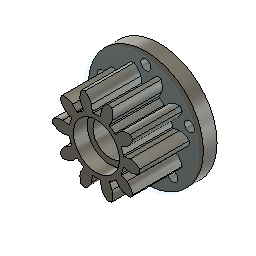
インナーギヤ v15 (Autodesk Fusion 360 design; units mm, degrees)
description: Spur Gear; Module: 1.580000; Num Teeth: 10; Pressure Angle: 20.000000; Backlash: 0.10 mm
Autodesk Fusion 360 part; units mm, degrees
(part 1 of 6)
sketch "スケッチ1" plane through (0, 0, 0) normal (0, 0, 1) x (1, 0, 0)
sketch "スケッチ2" plane through (0, 0, 0) normal (0, 0, -1) x (-1, 0, 0)
  circle A0 centre (0, 0) radius 5
  arc A1 (-5.434928, -4.325344) -> (-5.399704, -4.049062) centre (-5.559714, -4.169048) ccw
  line L0 (-5.434928, -4.325344) -> (-5.88157, -4.68194)
  spline S0 degree 5 poles (-5.88157, -4.68194) (-5.88496, -4.684646) (-5.891658, -4.690149) (-5.901465, -4.698676) (-5.914079, -4.710563) (-5.929217, -4.726135) (-5.943899, -4.742229) (-5.958299, -4.758658) (-5.972545, -4.775276) (-5.986688, -4.792027) (-6.000723, -4.808908) (-6.014614, -4.825957) (-6.028313, -4.84322) (-6.041787, -4.86073) (-6.05503, -4.87849) (-6.068059, -4.896482) (-6.080899, -4.914676) (-6.093581, -4.93304) (-6.106125, -4.951551) (-6.118538, -4.970199) (-6.13082, -4.988985) (-6.142963, -5.007914) (-6.15496, -5.026993) (-6.166806, -5.046226) (-6.178501, -5.06561) (-6.190051, -5.085142) (-6.20146, -5.104812) (-6.212734, -5.124615) (-6.22388, -5.144544) (-6.234897, -5.164595) (-6.245788, -5.184769) (-6.25655, -5.205064) (-6.267184, -5.225479) (-6.27769, -5.246016) (-6.288068, -5.266671) (-6.298319, -5.287442) (-6.308445, -5.308327) (-6.318449, -5.329324) (-6.32833, -5.35043) (-6.338091, -5.371643) (-6.347731, -5.392962) (-6.35725, -5.414386) (-6.36665, -5.435913) (-6.375931, -5.457544) (-6.385092, -5.479276) (-6.394135, -5.501107) (-6.40306, -5.523038) (-6.411868, -5.545065) (-6.420559, -5.567189) (-6.429134, -5.589407) (-6.437594, -5.611719) (-6.445937, -5.634123) (-6.454166, -5.656619) (-6.462279, -5.679205) (-6.470278, -5.701881) (-6.478163, -5.724646) (-6.485934, -5.747498) (-6.49359, -5.770436) (-6.501134, -5.79346) (-6.508564, -5.816568) (-6.515881, -5.839761) (-6.523086, -5.863036) (-6.530178, -5.886393) (-6.537157, -5.909831) (-6.544025, -5.93335) (-6.55078, -5.956947) (-6.557424, -5.980623) (-6.563955, -6.004376) (-6.570375, -6.028206) (-6.576684, -6.052112) (-6.582882, -6.076094) (-6.587751, -6.09534) (-6.591353, -6.109808) (-6.593732, -6.119468) (-6.594916, -6.124302) knots 0 0 0 0 0 0 0.01428571 0.02857143 0.04285714 0.05714286 0.07142857 0.08571429 0.1 0.11428571 0.12857143 0.14285714 0.15714286 0.17142857 0.18571429 0.2 0.21428571 0.22857143 0.24285714 0.25714286 0.27142857 0.28571429 0.3 0.31428571 0.32857143 0.34285714 0.35714286 0.37142857 0.38571429 0.4 0.41428571 0.42857143 0.44285714 0.45714286 0.47142857 0.48571429 0.5 0.51428571 0.52857143 0.54285714 0.55714286 0.57142857 0.58571429 0.6 0.61428571 0.62857143 0.64285714 0.65714286 0.67142857 0.68571429 0.7 0.71428571 0.72857143 0.74285714 0.75714286 0.77142857 0.78571429 0.8 0.81428571 0.82857143 0.84285714 0.85714286 0.87142857 0.88571429 0.9 0.91428571 0.92857143 0.94285714 0.95714286 0.97142857 0.98571429 1 1 1 1 1 1
  arc A2 (-6.594916, -6.124302) -> (-6.124302, -6.594916) centre (0, 0) ccw
  spline S1 degree 5 poles (-4.68194, -5.88157) (-4.684646, -5.88496) (-4.690149, -5.891658) (-4.698676, -5.901465) (-4.710563, -5.914079) (-4.726135, -5.929217) (-4.742229, -5.943899) (-4.758658, -5.958299) (-4.775276, -5.972545) (-4.792027, -5.986688) (-4.808908, -6.000723) (-4.825957, -6.014614) (-4.84322, -6.028313) (-4.86073, -6.041787) (-4.87849, -6.05503) (-4.896482, -6.068059) (-4.914676, -6.080899) (-4.93304, -6.093581) (-4.951551, -6.106125) (-4.970199, -6.118538) (-4.988985, -6.13082) (-5.007914, -6.142963) (-5.026993, -6.15496) (-5.046226, -6.166806) (-5.06561, -6.178501) (-5.085142, -6.190051) (-5.104812, -6.20146) (-5.124615, -6.212734) (-5.144544, -6.22388) (-5.164595, -6.234897) (-5.184769, -6.245788) (-5.205064, -6.25655) (-5.225479, -6.267184) (-5.246016, -6.27769) (-5.266671, -6.288068) (-5.287442, -6.298319) (-5.308327, -6.308445) (-5.329324, -6.318449) (-5.35043, -6.32833) (-5.371643, -6.338091) (-5.392962, -6.347731) (-5.414386, -6.35725) (-5.435913, -6.36665) (-5.457544, -6.375931) (-5.479276, -6.385092) (-5.501107, -6.394135) (-5.523038, -6.40306) (-5.545065, -6.411868) (-5.567189, -6.420559) (-5.589407, -6.429134) (-5.611719, -6.437594) (-5.634123, -6.445937) (-5.656619, -6.454166) (-5.679205, -6.462279) (-5.701881, -6.470278) (-5.724646, -6.478163) (-5.747498, -6.485934) (-5.770436, -6.49359) (-5.79346, -6.501134) (-5.816568, -6.508564) (-5.839761, -6.515881) (-5.863036, -6.523086) (-5.886393, -6.530178) (-5.909831, -6.537157) (-5.93335, -6.544025) (-5.956947, -6.55078) (-5.980623, -6.557424) (-6.004376, -6.563955) (-6.028206, -6.570375) (-6.052112, -6.576684) (-6.076094, -6.582882) (-6.09534, -6.587751) (-6.109808, -6.591353) (-6.119468, -6.593732) (-6.124302, -6.594916) knots 0 0 0 0 0 0 0.01428571 0.02857143 0.04285714 0.05714286 0.07142857 0.08571429 0.1 0.11428571 0.12857143 0.14285714 0.15714286 0.17142857 0.18571429 0.2 0.21428571 0.22857143 0.24285714 0.25714286 0.27142857 0.28571429 0.3 0.31428571 0.32857143 0.34285714 0.35714286 0.37142857 0.38571429 0.4 0.41428571 0.42857143 0.44285714 0.45714286 0.47142857 0.48571429 0.5 0.51428571 0.52857143 0.54285714 0.55714286 0.57142857 0.58571429 0.6 0.61428571 0.62857143 0.64285714 0.65714286 0.67142857 0.68571429 0.7 0.71428571 0.72857143 0.74285714 0.75714286 0.77142857 0.78571429 0.8 0.81428571 0.82857143 0.84285714 0.85714286 0.87142857 0.88571429 0.9 0.91428571 0.92857143 0.94285714 0.95714286 0.97142857 0.98571429 1 1 1 1 1 1
  line L1 (-4.68194, -5.88157) -> (-4.325344, -5.434928)
  arc A3 (-4.049062, -5.399704) -> (-4.325344, -5.434928) centre (-4.169048, -5.559714) ccw
  arc A4 (-4.049062, -5.399704) -> (-3.439167, -5.807222) centre (0, 0) ccw
  arc A5 (-3.365981, -6.075954) -> (-3.439167, -5.807222) centre (-3.54108, -5.979309) ccw
  line L2 (-3.365981, -6.075954) -> (-3.642161, -6.576327)
  spline S2 degree 5 poles (-3.642161, -6.576327) (-3.644257, -6.580125) (-3.64834, -6.587773) (-3.654137, -6.599403) (-3.661242, -6.615212) (-3.669269, -6.635392) (-3.676674, -6.655881) (-3.683691, -6.676569) (-3.690493, -6.697374) (-3.697149, -6.718261) (-3.703656, -6.739229) (-3.709965, -6.760296) (-3.716015, -6.781487) (-3.721762, -6.802821) (-3.727201, -6.824297) (-3.732353, -6.845905) (-3.737253, -6.867628) (-3.741942, -6.889448) (-3.746447, -6.91135) (-3.750779, -6.933329) (-3.754937, -6.955385) (-3.758912, -6.977519) (-3.762695, -6.999737) (-3.766279, -7.022039) (-3.769666, -7.044424) (-3.772862, -7.066888) (-3.775875, -7.089427) (-3.778713, -7.112037) (-3.781383, -7.134714) (-3.783889, -7.157456) (-3.78623, -7.180261) (-3.788407, -7.20313) (-3.790419, -7.226061) (-3.792266, -7.249054) (-3.79395, -7.272109) (-3.795472, -7.295222) (-3.796835, -7.318393) (-3.798041, -7.341619) (-3.799094, -7.3649) (-3.799994, -7.388233) (-3.800741, -7.411618) (-3.801338, -7.435054) (-3.801784, -7.458541) (-3.80208, -7.482076) (-3.802228, -7.505659) (-3.802228, -7.52929) (-3.802081, -7.552966) (-3.801789, -7.576688) (-3.801352, -7.600453) (-3.800772, -7.624262) (-3.800049, -7.648112) (-3.799184, -7.672004) (-3.798177, -7.695937) (-3.79703, -7.719909) (-3.795742, -7.74392) (-3.794315, -7.767969) (-3.792749, -7.792055) (-3.791045, -7.816177) (-3.789203, -7.840335) (-3.787225, -7.864528) (-3.78511, -7.888755) (-3.782859, -7.913015) (-3.780473, -7.937309) (-3.777952, -7.961634) (-3.775296, -7.98599) (-3.772507, -8.010377) (-3.769584, -8.034793) (-3.766529, -8.059237) (-3.763341, -8.08371) (-3.760021, -8.108211) (-3.756569, -8.132739) (-3.753703, -8.152383) (-3.751494, -8.167128) (-3.749995, -8.176964) (-3.749239, -8.181883) knots 0 0 0 0 0 0 0.01428571 0.02857143 0.04285714 0.05714286 0.07142857 0.08571429 0.1 0.11428571 0.12857143 0.14285714 0.15714286 0.17142857 0.18571429 0.2 0.21428571 0.22857143 0.24285714 0.25714286 0.27142857 0.28571429 0.3 0.31428571 0.32857143 0.34285714 0.35714286 0.37142857 0.38571429 0.4 0.41428571 0.42857143 0.44285714 0.45714286 0.47142857 0.48571429 0.5 0.51428571 0.52857143 0.54285714 0.55714286 0.57142857 0.58571429 0.6 0.61428571 0.62857143 0.64285714 0.65714286 0.67142857 0.68571429 0.7 0.71428571 0.72857143 0.74285714 0.75714286 0.77142857 0.78571429 0.8 0.81428571 0.82857143 0.84285714 0.85714286 0.87142857 0.88571429 0.9 0.91428571 0.92857143 0.94285714 0.95714286 0.97142857 0.98571429 1 1 1 1 1 1
  arc A6 (-3.749239, -8.181883) -> (-3.134352, -8.436577) centre (0, 0) ccw
  spline S3 degree 5 poles (-2.074769, -7.225563) (-2.075972, -7.22973) (-2.078493, -7.238025) (-2.082618, -7.250348) (-2.088772, -7.266551) (-2.097366, -7.286496) (-2.106617, -7.30622) (-2.116284, -7.32581) (-2.126186, -7.345331) (-2.136249, -7.364807) (-2.146475, -7.384235) (-2.15691, -7.403593) (-2.167616, -7.422855) (-2.178637, -7.442004) (-2.189978, -7.461035) (-2.201614, -7.479958) (-2.213509, -7.498784) (-2.225622, -7.517528) (-2.237924, -7.536201) (-2.250402, -7.554805) (-2.263058, -7.573341) (-2.275899, -7.591804) (-2.288935, -7.610188) (-2.30217, -7.628493) (-2.315604, -7.646716) (-2.329228, -7.66486) (-2.343036, -7.682929) (-2.357016, -7.700923) (-2.371163, -7.718847) (-2.385472, -7.736699) (-2.399942, -7.75448) (-2.414574, -7.77219) (-2.429366, -7.789828) (-2.444319, -7.807393) (-2.45943, -7.824885) (-2.474697, -7.842305) (-2.490117, -7.859653) (-2.505688, -7.876929) (-2.521405, -7.894135) (-2.537268, -7.911271) (-2.553276, -7.928335) (-2.569426, -7.945329) (-2.585717, -7.962252) (-2.60215, -7.979103) (-2.618722, -7.995884) (-2.635431, -8.012593) (-2.652276, -8.029231) (-2.669257, -8.045798) (-2.68637, -8.062294) (-2.703615, -8.078719) (-2.720992, -8.095073) (-2.738497, -8.111355) (-2.756132, -8.127566) (-2.773894, -8.143706) (-2.791783, -8.159773) (-2.809798, -8.175769) (-2.827936, -8.191694) (-2.846198, -8.207546) (-2.864583, -8.223326) (-2.883089, -8.239033) (-2.901715, -8.254669) (-2.920462, -8.270232) (-2.939327, -8.285723) (-2.95831, -8.30114) (-2.97741, -8.316485) (-2.996627, -8.331757) (-3.015958, -8.346955) (-3.035403, -8.362079) (-3.054963, -8.37713) (-3.074635, -8.392107) (-3.094419, -8.40701) (-3.110336, -8.418874) (-3.122325, -8.427738) (-3.130339, -8.433633) (-3.134352, -8.436577) knots 0 0 0 0 0 0 0.01428571 0.02857143 0.04285714 0.05714286 0.07142857 0.08571429 0.1 0.11428571 0.12857143 0.14285714 0.15714286 0.17142857 0.18571429 0.2 0.21428571 0.22857143 0.24285714 0.25714286 0.27142857 0.28571429 0.3 0.31428571 0.32857143 0.34285714 0.35714286 0.37142857 0.38571429 0.4 0.41428571 0.42857143 0.44285714 0.45714286 0.47142857 0.48571429 0.5 0.51428571 0.52857143 0.54285714 0.55714286 0.57142857 0.58571429 0.6 0.61428571 0.62857143 0.64285714 0.65714286 0.67142857 0.68571429 0.7 0.71428571 0.72857143 0.74285714 0.75714286 0.77142857 0.78571429 0.8 0.81428571 0.82857143 0.84285714 0.85714286 0.87142857 0.88571429 0.9 0.91428571 0.92857143 0.94285714 0.95714286 0.97142857 0.98571429 1 1 1 1 1 1
  line L3 (-2.074769, -7.225563) -> (-1.91624, -6.676457)
  arc A7 (-1.674468, -6.538185) -> (-1.91624, -6.676457) centre (-1.724088, -6.731931) ccw
  arc A8 (-1.674468, -6.538185) -> (-0.955048, -6.681286) centre (0, 0) ccw
  arc A9 (-0.784594, -6.901555) -> (-0.955048, -6.681286) centre (-0.983349, -6.879274) ccw
  line L4 (-0.784594, -6.901555) -> (-0.848267, -7.469529)
  spline S4 degree 5 poles (-0.848267, -7.469529) (-0.84875, -7.47384) (-0.849595, -7.482468) (-0.8505, -7.495431) (-0.851015, -7.512756) (-0.850708, -7.534471) (-0.849709, -7.556234) (-0.848274, -7.578033) (-0.846597, -7.599857) (-0.844753, -7.621702) (-0.84274, -7.643564) (-0.840507, -7.665441) (-0.837988, -7.687335) (-0.835133, -7.709243) (-0.831939, -7.731166) (-0.82843, -7.753101) (-0.824645, -7.775046) (-0.820626, -7.796999) (-0.816407, -7.818958) (-0.811998, -7.840922) (-0.807399, -7.86289) (-0.802601, -7.884861) (-0.797593, -7.906835) (-0.79237, -7.92881) (-0.786933, -7.950787) (-0.781289, -7.972765) (-0.775447, -7.994741) (-0.769417, -8.016717) (-0.763206, -8.038689) (-0.756818, -8.060658) (-0.750254, -8.082624) (-0.743513, -8.104585) (-0.736597, -8.126541) (-0.729504, -8.14849) (-0.722237, -8.170434) (-0.714798, -8.19237) (-0.70719, -8.214299) (-0.699417, -8.236219) (-0.69148, -8.25813) (-0.683382, -8.280032) (-0.675124, -8.301923) (-0.666706, -8.323804) (-0.65813, -8.345673) (-0.649398, -8.36753) (-0.640509, -8.389375) (-0.631466, -8.411206) (-0.62227, -8.433025) (-0.612922, -8.454829) (-0.603424, -8.476618) (-0.593777, -8.498392) (-0.583982, -8.52015) (-0.574039, -8.541893) (-0.563951, -8.563618) (-0.553717, -8.585326) (-0.543339, -8.607017) (-0.532817, -8.628689) (-0.522153, -8.650342) (-0.511347, -8.671976) (-0.500401, -8.693591) (-0.489315, -8.715185) (-0.47809, -8.736758) (-0.466726, -8.75831) (-0.455225, -8.779841) (-0.443587, -8.80135) (-0.431813, -8.822836) (-0.419903, -8.844299) (-0.40786, -8.865738) (-0.395682, -8.887153) (-0.383372, -8.908543) (-0.370928, -8.929908) (-0.358353, -8.951247) (-0.348188, -8.968299) (-0.340504, -8.981077) (-0.335355, -8.98959) (-0.332775, -8.993846) knots 0 0 0 0 0 0 0.01428571 0.02857143 0.04285714 0.05714286 0.07142857 0.08571429 0.1 0.11428571 0.12857143 0.14285714 0.15714286 0.17142857 0.18571429 0.2 0.21428571 0.22857143 0.24285714 0.25714286 0.27142857 0.28571429 0.3 0.31428571 0.32857143 0.34285714 0.35714286 0.37142857 0.38571429 0.4 0.41428571 0.42857143 0.44285714 0.45714286 0.47142857 0.48571429 0.5 0.51428571 0.52857143 0.54285714 0.55714286 0.57142857 0.58571429 0.6 0.61428571 0.62857143 0.64285714 0.65714286 0.67142857 0.68571429 0.7 0.71428571 0.72857143 0.74285714 0.75714286 0.77142857 0.78571429 0.8 0.81428571 0.82857143 0.84285714 0.85714286 0.87142857 0.88571429 0.9 0.91428571 0.92857143 0.94285714 0.95714286 0.97142857 0.98571429 1 1 1 1 1 1
  arc A10 (-0.332775, -8.993846) -> (0.332775, -8.993846) centre (0, 0) ccw
  spline S5 degree 5 poles (0.848267, -7.469529) (0.84875, -7.47384) (0.849595, -7.482468) (0.8505, -7.495431) (0.851015, -7.512756) (0.850708, -7.534471) (0.849709, -7.556234) (0.848274, -7.578033) (0.846597, -7.599857) (0.844753, -7.621702) (0.84274, -7.643564) (0.840507, -7.665441) (0.837988, -7.687335) (0.835133, -7.709243) (0.831939, -7.731166) (0.82843, -7.753101) (0.824645, -7.775046) (0.820626, -7.796999) (0.816407, -7.818958) (0.811998, -7.840922) (0.807399, -7.86289) (0.802601, -7.884861) (0.797593, -7.906835) (0.79237, -7.92881) (0.786933, -7.950787) (0.781289, -7.972765) (0.775447, -7.994741) (0.769417, -8.016717) (0.763206, -8.038689) (0.756818, -8.060658) (0.750254, -8.082624) (0.743513, -8.104585) (0.736597, -8.126541) (0.729504, -8.14849) (0.722237, -8.170434) (0.714798, -8.19237) (0.70719, -8.214299) (0.699417, -8.236219) (0.69148, -8.25813) (0.683382, -8.280032) (0.675124, -8.301923) (0.666706, -8.323804) (0.65813, -8.345673) (0.649398, -8.36753) (0.640509, -8.389375) (0.631466, -8.411206) (0.62227, -8.433025) (0.612922, -8.454829) (0.603424, -8.476618) (0.593777, -8.498392) (0.583982, -8.52015) (0.574039, -8.541893) (0.563951, -8.563618) (0.553717, -8.585326) (0.543339, -8.607017) (0.532817, -8.628689) (0.522153, -8.650342) (0.511347, -8.671976) (0.500401, -8.693591) (0.489315, -8.715185) (0.47809, -8.736758) (0.466726, -8.75831) (0.455225, -8.779841) (0.443587, -8.80135) (0.431813, -8.822836) (0.419903, -8.844299) (0.40786, -8.865738) (0.395682, -8.887153) (0.383372, -8.908543) (0.370928, -8.929908) (0.358353, -8.951247) (0.348188, -8.968299) (0.340504, -8.981077) (0.335355, -8.98959) (0.332775, -8.993846) knots 0 0 0 0 0 0 0.01428571 0.02857143 0.04285714 0.05714286 0.07142857 0.08571429 0.1 0.11428571 0.12857143 0.14285714 0.15714286 0.17142857 0.18571429 0.2 0.21428571 0.22857143 0.24285714 0.25714286 0.27142857 0.28571429 0.3 0.31428571 0.32857143 0.34285714 0.35714286 0.37142857 0.38571429 0.4 0.41428571 0.42857143 0.44285714 0.45714286 0.47142857 0.48571429 0.5 0.51428571 0.52857143 0.54285714 0.55714286 0.57142857 0.58571429 0.6 0.61428571 0.62857143 0.64285714 0.65714286 0.67142857 0.68571429 0.7 0.71428571 0.72857143 0.74285714 0.75714286 0.77142857 0.78571429 0.8 0.81428571 0.82857143 0.84285714 0.85714286 0.87142857 0.88571429 0.9 0.91428571 0.92857143 0.94285714 0.95714286 0.97142857 0.98571429 1 1 1 1 1 1
  line L5 (0.848267, -7.469529) -> (0.784594, -6.901555)
  arc A11 (0.955048, -6.681286) -> (0.784594, -6.901555) centre (0.983349, -6.879274) ccw
  arc A12 (0.955048, -6.681286) -> (1.674468, -6.538185) centre (0, 0) ccw
  arc A13 (1.91624, -6.676457) -> (1.674468, -6.538185) centre (1.724088, -6.731931) ccw
  line L6 (1.91624, -6.676457) -> (2.074769, -7.225563)
  spline S6 degree 5 poles (2.074769, -7.225563) (2.075972, -7.22973) (2.078493, -7.238025) (2.082618, -7.250348) (2.088772, -7.266551) (2.097366, -7.286496) (2.106617, -7.30622) (2.116284, -7.32581) (2.126186, -7.345331) (2.136249, -7.364807) (2.146475, -7.384235) (2.15691, -7.403593) (2.167616, -7.422855) (2.178637, -7.442004) (2.189978, -7.461035) (2.201614, -7.479958) (2.213509, -7.498784) (2.225622, -7.517528) (2.237924, -7.536201) (2.250402, -7.554805) (2.263058, -7.573341) (2.275899, -7.591804) (2.288935, -7.610188) (2.30217, -7.628493) (2.315604, -7.646716) (2.329228, -7.66486) (2.343036, -7.682929) (2.357016, -7.700923) (2.371163, -7.718847) (2.385472, -7.736699) (2.399942, -7.75448) (2.414574, -7.77219) (2.429366, -7.789828) (2.444319, -7.807393) (2.45943, -7.824885) (2.474697, -7.842305) (2.490117, -7.859653) (2.505688, -7.876929) (2.521405, -7.894135) (2.537268, -7.911271) (2.553276, -7.928335) (2.569426, -7.945329) (2.585717, -7.962252) (2.60215, -7.979103) (2.618722, -7.995884) (2.635431, -8.012593) (2.652276, -8.029231) (2.669257, -8.045798) (2.68637, -8.062294) (2.703615, -8.078719) (2.720992, -8.095073) (2.738497, -8.111355) (2.756132, -8.127566) (2.773894, -8.143706) (2.791783, -8.159773) (2.809798, -8.175769) (2.827936, -8.191694) (2.846198, -8.207546) (2.864583, -8.223326) (2.883089, -8.239033) (2.901715, -8.254669) (2.920462, -8.270232) (2.939327, -8.285723) (2.95831, -8.30114) (2.97741, -8.316485) (2.996627, -8.331757) (3.015958, -8.346955) (3.035403, -8.362079) (3.054963, -8.37713) (3.074635, -8.392107) (3.094419, -8.40701) (3.110336, -8.418874) (3.122325, -8.427738) (3.130339, -8.433633) (3.134352, -8.436577) knots 0 0 0 0 0 0 0.01428571 0.02857143 0.04285714 0.05714286 0.07142857 0.08571429 0.1 0.11428571 0.12857143 0.14285714 0.15714286 0.17142857 0.18571429 0.2 0.21428571 0.22857143 0.24285714 0.25714286 0.27142857 0.28571429 0.3 0.31428571 0.32857143 0.34285714 0.35714286 0.37142857 0.38571429 0.4 0.41428571 0.42857143 0.44285714 0.45714286 0.47142857 0.48571429 0.5 0.51428571 0.52857143 0.54285714 0.55714286 0.57142857 0.58571429 0.6 0.61428571 0.62857143 0.64285714 0.65714286 0.67142857 0.68571429 0.7 0.71428571 0.72857143 0.74285714 0.75714286 0.77142857 0.78571429 0.8 0.81428571 0.82857143 0.84285714 0.85714286 0.87142857 0.88571429 0.9 0.91428571 0.92857143 0.94285714 0.95714286 0.97142857 0.98571429 1 1 1 1 1 1
  arc A14 (3.134352, -8.436577) -> (3.749239, -8.181883) centre (0, 0) ccw
  spline S7 degree 5 poles (3.642161, -6.576327) (3.644257, -6.580125) (3.64834, -6.587773) (3.654137, -6.599403) (3.661242, -6.615212) (3.669269, -6.635392) (3.676674, -6.655881) (3.683691, -6.676569) (3.690493, -6.697374) (3.697149, -6.718261) (3.703656, -6.739229) (3.709965, -6.760296) (3.716015, -6.781487) (3.721762, -6.802821) (3.727201, -6.824297) (3.732353, -6.845905) (3.737253, -6.867628) (3.741942, -6.889448) (3.746447, -6.91135) (3.750779, -6.933329) (3.754937, -6.955385) (3.758912, -6.977519) (3.762695, -6.999737) (3.766279, -7.022039) (3.769666, -7.044424) (3.772862, -7.066888) (3.775875, -7.089427) (3.778713, -7.112037) (3.781383, -7.134714) (3.783889, -7.157456) (3.78623, -7.180261) (3.788407, -7.20313) (3.790419, -7.226061) (3.792266, -7.249054) (3.79395, -7.272109) (3.795472, -7.295222) (3.796835, -7.318393) (3.798041, -7.341619) (3.799094, -7.3649) (3.799994, -7.388233) (3.800741, -7.411618) (3.801338, -7.435054) (3.801784, -7.458541) (3.80208, -7.482076) (3.802228, -7.505659) (3.802228, -7.52929) (3.802081, -7.552966) (3.801789, -7.576688) (3.801352, -7.600453) (3.800772, -7.624262) (3.800049, -7.648112) (3.799184, -7.672004) (3.798177, -7.695937) (3.79703, -7.719909) (3.795742, -7.74392) (3.794315, -7.767969) (3.792749, -7.792055) (3.791045, -7.816177) (3.789203, -7.840335) (3.787225, -7.864528) (3.78511, -7.888755) (3.782859, -7.913015) (3.780473, -7.937309) (3.777952, -7.961634) (3.775296, -7.98599) (3.772507, -8.010377) (3.769584, -8.034793) (3.766529, -8.059237) (3.763341, -8.08371) (3.760021, -8.108211) (3.756569, -8.132739) (3.753703, -8.152383) (3.751494, -8.167128) (3.749995, -8.176964) (3.749239, -8.181883) knots 0 0 0 0 0 0 0.01428571 0.02857143 0.04285714 0.05714286 0.07142857 0.08571429 0.1 0.11428571 0.12857143 0.14285714 0.15714286 0.17142857 0.18571429 0.2 0.21428571 0.22857143 0.24285714 0.25714286 0.27142857 0.28571429 0.3 0.31428571 0.32857143 0.34285714 0.35714286 0.37142857 0.38571429 0.4 0.41428571 0.42857143 0.44285714 0.45714286 0.47142857 0.48571429 0.5 0.51428571 0.52857143 0.54285714 0.55714286 0.57142857 0.58571429 0.6 0.61428571 0.62857143 0.64285714 0.65714286 0.67142857 0.68571429 0.7 0.71428571 0.72857143 0.74285714 0.75714286 0.77142857 0.78571429 0.8 0.81428571 0.82857143 0.84285714 0.85714286 0.87142857 0.88571429 0.9 0.91428571 0.92857143 0.94285714 0.95714286 0.97142857 0.98571429 1 1 1 1 1 1
  line L7 (3.642161, -6.576327) -> (3.365981, -6.075954)
  arc A15 (3.439167, -5.807222) -> (3.365981, -6.075954) centre (3.54108, -5.979309) ccw
  arc A16 (3.439167, -5.807222) -> (4.049062, -5.399704) centre (0, 0) ccw
  arc A17 (4.325344, -5.434928) -> (4.049062, -5.399704) centre (4.169048, -5.559714) ccw
  line L8 (4.325344, -5.434928) -> (4.68194, -5.88157)
  spline S8 degree 5 poles (4.68194, -5.88157) (4.684646, -5.88496) (4.690149, -5.891658) (4.698676, -5.901465) (4.710563, -5.914079) (4.726135, -5.929217) (4.742229, -5.943899) (4.758658, -5.958299) (4.775276, -5.972545) (4.792027, -5.986688) (4.808908, -6.000723) (4.825957, -6.014614) (4.84322, -6.028313) (4.86073, -6.041787) (4.87849, -6.05503) (4.896482, -6.068059) (4.914676, -6.080899) (4.93304, -6.093581) (4.951551, -6.106125) (4.970199, -6.118538) (4.988985, -6.13082) (5.007914, -6.142963) (5.026993, -6.15496) (5.046226, -6.166806) (5.06561, -6.178501) (5.085142, -6.190051) (5.104812, -6.20146) (5.124615, -6.212734) (5.144544, -6.22388) (5.164595, -6.234897) (5.184769, -6.245788) (5.205064, -6.25655) (5.225479, -6.267184) (5.246016, -6.27769) (5.266671, -6.288068) (5.287442, -6.298319) (5.308327, -6.308445) (5.329324, -6.318449) (5.35043, -6.32833) (5.371643, -6.338091) (5.392962, -6.347731) (5.414386, -6.35725) (5.435913, -6.36665) (5.457544, -6.375931) (5.479276, -6.385092) (5.501107, -6.394135) (5.523038, -6.40306) (5.545065, -6.411868) (5.567189, -6.420559) (5.589407, -6.429134) (5.611719, -6.437594) (5.634123, -6.445937) (5.656619, -6.454166) (5.679205, -6.462279) (5.701881, -6.470278) (5.724646, -6.478163) (5.747498, -6.485934) (5.770436, -6.49359) (5.79346, -6.501134) (5.816568, -6.508564) (5.839761, -6.515881) (5.863036, -6.523086) (5.886393, -6.530178) (5.909831, -6.537157) (5.93335, -6.544025) (5.956947, -6.55078) (5.980623, -6.557424) (6.004376, -6.563955) (6.028206, -6.570375) (6.052112, -6.576684) (6.076094, -6.582882) (6.09534, -6.587751) (6.109808, -6.591353) (6.119468, -6.593732) (6.124302, -6.594916) knots 0 0 0 0 0 0 0.01428571 0.02857143 0.04285714 0.05714286 0.07142857 0.08571429 0.1 0.11428571 0.12857143 0.14285714 0.15714286 0.17142857 0.18571429 0.2 0.21428571 0.22857143 0.24285714 0.25714286 0.27142857 0.28571429 0.3 0.31428571 0.32857143 0.34285714 0.35714286 0.37142857 0.38571429 0.4 0.41428571 0.42857143 0.44285714 0.45714286 0.47142857 0.48571429 0.5 0.51428571 0.52857143 0.54285714 0.55714286 0.57142857 0.58571429 0.6 0.61428571 0.62857143 0.64285714 0.65714286 0.67142857 0.68571429 0.7 0.71428571 0.72857143 0.74285714 0.75714286 0.77142857 0.78571429 0.8 0.81428571 0.82857143 0.84285714 0.85714286 0.87142857 0.88571429 0.9 0.91428571 0.92857143 0.94285714 0.95714286 0.97142857 0.98571429 1 1 1 1 1 1
  arc A18 (6.124302, -6.594916) -> (6.594916, -6.124302) centre (0, 0) ccw
  spline S9 degree 5 poles (5.88157, -4.68194) (5.88496, -4.684646) (5.891658, -4.690149) (5.901465, -4.698676) (5.914079, -4.710563) (5.929217, -4.726135) (5.943899, -4.742229) (5.958299, -4.758658) (5.972545, -4.775276) (5.986688, -4.792027) (6.000723, -4.808908) (6.014614, -4.825957) (6.028313, -4.84322) (6.041787, -4.86073) (6.05503, -4.87849) (6.068059, -4.896482) (6.080899, -4.914676) (6.093581, -4.93304) (6.106125, -4.951551) (6.118538, -4.970199) (6.13082, -4.988985) (6.142963, -5.007914) (6.15496, -5.026993) (6.166806, -5.046226) (6.178501, -5.06561) (6.190051, -5.085142) (6.20146, -5.104812) (6.212734, -5.124615) (6.22388, -5.144544) (6.234897, -5.164595) (6.245788, -5.184769) (6.25655, -5.205064) (6.267184, -5.225479) (6.27769, -5.246016) (6.288068, -5.266671) (6.298319, -5.287442) (6.308445, -5.308327) (6.318449, -5.329324) (6.32833, -5.35043) (6.338091, -5.371643) (6.347731, -5.392962) (6.35725, -5.414386) (6.36665, -5.435913) (6.375931, -5.457544) (6.385092, -5.479276) (6.394135, -5.501107) (6.40306, -5.523038) (6.411868, -5.545065) (6.420559, -5.567189) (6.429134, -5.589407) (6.437594, -5.611719) (6.445937, -5.634123) (6.454166, -5.656619) (6.462279, -5.679205) (6.470278, -5.701881) (6.478163, -5.724646) (6.485934, -5.747498) (6.49359, -5.770436) (6.501134, -5.79346) (6.508564, -5.816568) (6.515881, -5.839761) (6.523086, -5.863036) (6.530178, -5.886393) (6.537157, -5.909831) (6.544025, -5.93335) (6.55078, -5.956947) (6.557424, -5.980623) (6.563955, -6.004376) (6.570375, -6.028206) (6.576684, -6.052112) (6.582882, -6.076094) (6.587751, -6.09534) (6.591353, -6.109808) (6.593732, -6.119468) (6.594916, -6.124302) knots 0 0 0 0 0 0 0.01428571 0.02857143 0.04285714 0.05714286 0.07142857 0.08571429 0.1 0.11428571 0.12857143 0.14285714 0.15714286 0.17142857 0.18571429 0.2 0.21428571 0.22857143 0.24285714 0.25714286 0.27142857 0.28571429 0.3 0.31428571 0.32857143 0.34285714 0.35714286 0.37142857 0.38571429 0.4 0.41428571 0.42857143 0.44285714 0.45714286 0.47142857 0.48571429 0.5 0.51428571 0.52857143 0.54285714 0.55714286 0.57142857 0.58571429 0.6 0.61428571 0.62857143 0.64285714 0.65714286 0.67142857 0.68571429 0.7 0.71428571 0.72857143 0.74285714 0.75714286 0.77142857 0.78571429 0.8 0.81428571 0.82857143 0.84285714 0.85714286 0.87142857 0.88571429 0.9 0.91428571 0.92857143 0.94285714 0.95714286 0.97142857 0.98571429 1 1 1 1 1 1
  line L9 (5.88157, -4.68194) -> (5.434928, -4.325344)
  arc A19 (5.399704, -4.049062) -> (5.434928, -4.325344) centre (5.559714, -4.169048) ccw
  arc A20 (5.399704, -4.049062) -> (5.807222, -3.439167) centre (0, 0) ccw
  arc A21 (6.075954, -3.365981) -> (5.807222, -3.439167) centre (5.979309, -3.54108) ccw
  line L10 (6.075954, -3.365981) -> (6.576327, -3.642161)
  spline S10 degree 5 poles (6.576327, -3.642161) (6.580125, -3.644257) (6.587773, -3.64834) (6.599403, -3.654137) (6.615212, -3.661242) (6.635392, -3.669269) (6.655881, -3.676674) (6.676569, -3.683691) (6.697374, -3.690493) (6.718261, -3.697149) (6.739229, -3.703656) (6.760296, -3.709965) (6.781487, -3.716015) (6.802821, -3.721762) (6.824297, -3.727201) (6.845905, -3.732353) (6.867628, -3.737253) (6.889448, -3.741942) (6.91135, -3.746447) (6.933329, -3.750779) (6.955385, -3.754937) (6.977519, -3.758912) (6.999737, -3.762695) (7.022039, -3.766279) (7.044424, -3.769666) (7.066888, -3.772862) (7.089427, -3.775875) (7.112037, -3.778713) (7.134714, -3.781383) (7.157456, -3.783889) (7.180261, -3.78623) (7.20313, -3.788407) (7.226061, -3.790419) (7.249054, -3.792266) (7.272109, -3.79395) (7.295222, -3.795472) (7.318393, -3.796835) (7.341619, -3.798041) (7.3649, -3.799094) (7.388233, -3.799994) (7.411618, -3.800741) (7.435054, -3.801338) (7.458541, -3.801784) (7.482076, -3.80208) (7.505659, -3.802228) (7.52929, -3.802228) (7.552966, -3.802081) (7.576688, -3.801789) (7.600453, -3.801352) (7.624262, -3.800772) (7.648112, -3.800049) (7.672004, -3.799184) (7.695937, -3.798177) (7.719909, -3.79703) (7.74392, -3.795742) (7.767969, -3.794315) (7.792055, -3.792749) (7.816177, -3.791045) (7.840335, -3.789203) (7.864528, -3.787225) (7.888755, -3.78511) (7.913015, -3.782859) (7.937309, -3.780473) (7.961634, -3.777952) (7.98599, -3.775296) (8.010377, -3.772507) (8.034793, -3.769584) (8.059237, -3.766529) (8.08371, -3.763341) (8.108211, -3.760021) (8.132739, -3.756569) (8.152383, -3.753703) (8.167128, -3.751494) (8.176964, -3.749995) (8.181883, -3.749239) knots 0 0 0 0 0 0 0.01428571 0.02857143 0.04285714 0.05714286 0.07142857 0.08571429 0.1 0.11428571 0.12857143 0.14285714 0.15714286 0.17142857 0.18571429 0.2 0.21428571 0.22857143 0.24285714 0.25714286 0.27142857 0.28571429 0.3 0.31428571 0.32857143 0.34285714 0.35714286 0.37142857 0.38571429 0.4 0.41428571 0.42857143 0.44285714 0.45714286 0.47142857 0.48571429 0.5 0.51428571 0.52857143 0.54285714 0.55714286 0.57142857 0.58571429 0.6 0.61428571 0.62857143 0.64285714 0.65714286 0.67142857 0.68571429 0.7 0.71428571 0.72857143 0.74285714 0.75714286 0.77142857 0.78571429 0.8 0.81428571 0.82857143 0.84285714 0.85714286 0.87142857 0.88571429 0.9 0.91428571 0.92857143 0.94285714 0.95714286 0.97142857 0.98571429 1 1 1 1 1 1
  arc A22 (8.181883, -3.749239) -> (8.436577, -3.134352) centre (0, 0) ccw
  spline S11 degree 5 poles (7.225563, -2.074769) (7.22973, -2.075972) (7.238025, -2.078493) (7.250348, -2.082618) (7.266551, -2.088772) (7.286496, -2.097366) (7.30622, -2.106617) (7.32581, -2.116284) (7.345331, -2.126186) (7.364807, -2.136249) (7.384235, -2.146475) (7.403593, -2.15691) (7.422855, -2.167616) (7.442004, -2.178637) (7.461035, -2.189978) (7.479958, -2.201614) (7.498784, -2.213509) (7.517528, -2.225622) (7.536201, -2.237924) (7.554805, -2.250402) (7.573341, -2.263058) (7.591804, -2.275899) (7.610188, -2.288935) (7.628493, -2.30217) (7.646716, -2.315604) (7.66486, -2.329228) (7.682929, -2.343036) (7.700923, -2.357016) (7.718847, -2.371163) (7.736699, -2.385472) (7.75448, -2.399942) (7.77219, -2.414574) (7.789828, -2.429366) (7.807393, -2.444319) (7.824885, -2.45943) (7.842305, -2.474697) (7.859653, -2.490117) (7.876929, -2.505688) (7.894135, -2.521405) (7.911271, -2.537268) (7.928335, -2.553276) (7.945329, -2.569426) (7.962252, -2.585717) (7.979103, -2.60215) (7.995884, -2.618722) (8.012593, -2.635431) (8.029231, -2.652276) (8.045798, -2.669257) (8.062294, -2.68637) (8.078719, -2.703615) (8.095073, -2.720992) (8.111355, -2.738497) (8.127566, -2.756132) (8.143706, -2.773894) (8.159773, -2.791783) (8.175769, -2.809798) (8.191694, -2.827936) (8.207546, -2.846198) (8.223326, -2.864583) (8.239033, -2.883089) (8.254669, -2.901715) (8.270232, -2.920462) (8.285723, -2.939327) (8.30114, -2.95831) (8.316485, -2.97741) (8.331757, -2.996627) (8.346955, -3.015958) (8.362079, -3.035403) (8.37713, -3.054963) (8.392107, -3.074635) (8.40701, -3.094419) (8.418874, -3.110336) (8.427738, -3.122325) (8.433633, -3.130339) (8.436577, -3.134352) knots 0 0 0 0 0 0 0.01428571 0.02857143 0.04285714 0.05714286 0.07142857 0.08571429 0.1 0.11428571 0.12857143 0.14285714 0.15714286 0.17142857 0.18571429 0.2 0.21428571 0.22857143 0.24285714 0.25714286 0.27142857 0.28571429 0.3 0.31428571 0.32857143 0.34285714 0.35714286 0.37142857 0.38571429 0.4 0.41428571 0.42857143 0.44285714 0.45714286 0.47142857 0.48571429 0.5 0.51428571 0.52857143 0.54285714 0.55714286 0.57142857 0.58571429 0.6 0.61428571 0.62857143 0.64285714 0.65714286 0.67142857 0.68571429 0.7 0.71428571 0.72857143 0.74285714 0.75714286 0.77142857 0.78571429 0.8 0.81428571 0.82857143 0.84285714 0.85714286 0.87142857 0.88571429 0.9 0.91428571 0.92857143 0.94285714 0.95714286 0.97142857 0.98571429 1 1 1 1 1 1
  line L11 (7.225563, -2.074769) -> (6.676457, -1.91624)
  arc A23 (6.538185, -1.674468) -> (6.676457, -1.91624) centre (6.731931, -1.724088) ccw
  arc A24 (6.538185, -1.674468) -> (6.681286, -0.955048) centre (0, 0) ccw
  arc A25 (6.901555, -0.784594) -> (6.681286, -0.955048) centre (6.879274, -0.983349) ccw
  line L12 (6.901555, -0.784594) -> (7.469529, -0.848267)
  spline S12 degree 5 poles (7.469529, -0.848267) (7.47384, -0.84875) (7.482468, -0.849595) (7.495431, -0.8505) (7.512756, -0.851015) (7.534471, -0.850708) (7.556234, -0.849709) (7.578033, -0.848274) (7.599857, -0.846597) (7.621702, -0.844753) (7.643564, -0.84274) (7.665441, -0.840507) (7.687335, -0.837988) (7.709243, -0.835133) (7.731166, -0.831939) (7.753101, -0.82843) (7.775046, -0.824645) (7.796999, -0.820626) (7.818958, -0.816407) (7.840922, -0.811998) (7.86289, -0.807399) (7.884861, -0.802601) (7.906835, -0.797593) (7.92881, -0.79237) (7.950787, -0.786933) (7.972765, -0.781289) (7.994741, -0.775447) (8.016717, -0.769417) (8.038689, -0.763206) (8.060658, -0.756818) (8.082624, -0.750254) (8.104585, -0.743513) (8.126541, -0.736597) (8.14849, -0.729504) (8.170434, -0.722237) (8.19237, -0.714798) (8.214299, -0.70719) (8.236219, -0.699417) (8.25813, -0.69148) (8.280032, -0.683382) (8.301923, -0.675124) (8.323804, -0.666706) (8.345673, -0.65813) (8.36753, -0.649398) (8.389375, -0.640509) (8.411206, -0.631466) (8.433025, -0.62227) (8.454829, -0.612922) (8.476618, -0.603424) (8.498392, -0.593777) (8.52015, -0.583982) (8.541893, -0.574039) (8.563618, -0.563951) (8.585326, -0.553717) (8.607017, -0.543339) (8.628689, -0.532817) (8.650342, -0.522153) (8.671976, -0.511347) (8.693591, -0.500401) (8.715185, -0.489315) (8.736758, -0.47809) (8.75831, -0.466726) (8.779841, -0.455225) (8.80135, -0.443587) (8.822836, -0.431813) (8.844299, -0.419903) (8.865738, -0.40786) (8.887153, -0.395682) (8.908543, -0.383372) (8.929908, -0.370928) (8.951247, -0.358353) (8.968299, -0.348188) (8.981077, -0.340504) (8.98959, -0.335355) (8.993846, -0.332775) knots 0 0 0 0 0 0 0.01428571 0.02857143 0.04285714 0.05714286 0.07142857 0.08571429 0.1 0.11428571 0.12857143 0.14285714 0.15714286 0.17142857 0.18571429 0.2 0.21428571 0.22857143 0.24285714 0.25714286 0.27142857 0.28571429 0.3 0.31428571 0.32857143 0.34285714 0.35714286 0.37142857 0.38571429 0.4 0.41428571 0.42857143 0.44285714 0.45714286 0.47142857 0.48571429 0.5 0.51428571 0.52857143 0.54285714 0.55714286 0.57142857 0.58571429 0.6 0.61428571 0.62857143 0.64285714 0.65714286 0.67142857 0.68571429 0.7 0.71428571 0.72857143 0.74285714 0.75714286 0.77142857 0.78571429 0.8 0.81428571 0.82857143 0.84285714 0.85714286 0.87142857 0.88571429 0.9 0.91428571 0.92857143 0.94285714 0.95714286 0.97142857 0.98571429 1 1 1 1 1 1
  arc A26 (8.993846, -0.332775) -> (8.993846, 0.332775) centre (0, 0) ccw
  spline S13 degree 5 poles (7.469529, 0.848267) (7.47384, 0.84875) (7.482468, 0.849595) (7.495431, 0.8505) (7.512756, 0.851015) (7.534471, 0.850708) (7.556234, 0.849709) (7.578033, 0.848274) (7.599857, 0.846597) (7.621702, 0.844753) (7.643564, 0.84274) (7.665441, 0.840507) (7.687335, 0.837988) (7.709243, 0.835133) (7.731166, 0.831939) (7.753101, 0.82843) (7.775046, 0.824645) (7.796999, 0.820626) (7.818958, 0.816407) (7.840922, 0.811998) (7.86289, 0.807399) (7.884861, 0.802601) (7.906835, 0.797593) (7.92881, 0.79237) (7.950787, 0.786933) (7.972765, 0.781289) (7.994741, 0.775447) (8.016717, 0.769417) (8.038689, 0.763206) (8.060658, 0.756818) (8.082624, 0.750254) (8.104585, 0.743513) (8.126541, 0.736597) (8.14849, 0.729504) (8.170434, 0.722237) (8.19237, 0.714798) (8.214299, 0.70719) (8.236219, 0.699417) (8.25813, 0.69148) (8.280032, 0.683382) (8.301923, 0.675124) (8.323804, 0.666706) (8.345673, 0.65813) (8.36753, 0.649398) (8.389375, 0.640509) (8.411206, 0.631466) (8.433025, 0.62227) (8.454829, 0.612922) (8.476618, 0.603424) (8.498392, 0.593777) (8.52015, 0.583982) (8.541893, 0.574039) (8.563618, 0.563951) (8.585326, 0.553717) (8.607017, 0.543339) (8.628689, 0.532817) (8.650342, 0.522153) (8.671976, 0.511347) (8.693591, 0.500401) (8.715185, 0.489315) (8.736758, 0.47809) (8.75831, 0.466726) (8.779841, 0.455225) (8.80135, 0.443587) (8.822836, 0.431813) (8.844299, 0.419903) (8.865738, 0.40786) (8.887153, 0.395682) (8.908543, 0.383372) (8.929908, 0.370928) (8.951247, 0.358353) (8.968299, 0.348188) (8.981077, 0.340504) (8.98959, 0.335355) (8.993846, 0.332775) knots 0 0 0 0 0 0 0.01428571 0.02857143 0.04285714 0.05714286 0.07142857 0.08571429 0.1 0.11428571 0.12857143 0.14285714 0.15714286 0.17142857 0.18571429 0.2 0.21428571 0.22857143 0.24285714 0.25714286 0.27142857 0.28571429 0.3 0.31428571 0.32857143 0.34285714 0.35714286 0.37142857 0.38571429 0.4 0.41428571 0.42857143 0.44285714 0.45714286 0.47142857 0.48571429 0.5 0.51428571 0.52857143 0.54285714 0.55714286 0.57142857 0.58571429 0.6 0.61428571 0.62857143 0.64285714 0.65714286 0.67142857 0.68571429 0.7 0.71428571 0.72857143 0.74285714 0.75714286 0.77142857 0.78571429 0.8 0.81428571 0.82857143 0.84285714 0.85714286 0.87142857 0.88571429 0.9 0.91428571 0.92857143 0.94285714 0.95714286 0.97142857 0.98571429 1 1 1 1 1 1
  line L13 (7.469529, 0.848267) -> (6.901555, 0.784594)
  arc A27 (6.681286, 0.955048) -> (6.901555, 0.784594) centre (6.879274, 0.983349) ccw
  arc A28 (6.681286, 0.955048) -> (6.538185, 1.674468) centre (0, 0) ccw
  arc A29 (6.676457, 1.91624) -> (6.538185, 1.674468) centre (6.731931, 1.724088) ccw
  line L14 (6.676457, 1.91624) -> (7.225563, 2.074769)
  spline S14 degree 5 poles (7.225563, 2.074769) (7.22973, 2.075972) (7.238025, 2.078493) (7.250348, 2.082618) (7.266551, 2.088772) (7.286496, 2.097366) (7.30622, 2.106617) (7.32581, 2.116284) (7.345331, 2.126186) (7.364807, 2.136249) (7.384235, 2.146475) (7.403593, 2.15691) (7.422855, 2.167616) (7.442004, 2.178637) (7.461035, 2.189978) (7.479958, 2.201614) (7.498784, 2.213509) (7.517528, 2.225622) (7.536201, 2.237924) (7.554805, 2.250402) (7.573341, 2.263058) (7.591804, 2.275899) (7.610188, 2.288935) (7.628493, 2.30217) (7.646716, 2.315604) (7.66486, 2.329228) (7.682929, 2.343036) (7.700923, 2.357016) (7.718847, 2.371163) (7.736699, 2.385472) (7.75448, 2.399942) (7.77219, 2.414574) (7.789828, 2.429366) (7.807393, 2.444319) (7.824885, 2.45943) (7.842305, 2.474697) (7.859653, 2.490117) (7.876929, 2.505688) (7.894135, 2.521405) (7.911271, 2.537268) (7.928335, 2.553276) (7.945329, 2.569426) (7.962252, 2.585717) (7.979103, 2.60215) (7.995884, 2.618722) (8.012593, 2.635431) (8.029231, 2.652276) (8.045798, 2.669257) (8.062294, 2.68637) (8.078719, 2.703615) (8.095073, 2.720992) (8.111355, 2.738497) (8.127566, 2.756132) (8.143706, 2.773894) (8.159773, 2.791783) (8.175769, 2.809798) (8.191694, 2.827936) (8.207546, 2.846198) (8.223326, 2.864583) (8.239033, 2.883089) (8.254669, 2.901715) (8.270232, 2.920462) (8.285723, 2.939327) (8.30114, 2.95831) (8.316485, 2.97741) (8.331757, 2.996627) (8.346955, 3.015958) (8.362079, 3.035403) (8.37713, 3.054963) (8.392107, 3.074635) (8.40701, 3.094419) (8.418874, 3.110336) (8.427738, 3.122325) (8.433633, 3.130339) (8.436577, 3.134352) knots 0 0 0 0 0 0 0.01428571 0.02857143 0.04285714 0.05714286 0.07142857 0.08571429 0.1 0.11428571 0.12857143 0.14285714 0.15714286 0.17142857 0.18571429 0.2 0.21428571 0.22857143 0.24285714 0.25714286 0.27142857 0.28571429 0.3 0.31428571 0.32857143 0.34285714 0.35714286 0.37142857 0.38571429 0.4 0.41428571 0.42857143 0.44285714 0.45714286 0.47142857 0.48571429 0.5 0.51428571 0.52857143 0.54285714 0.55714286 0.57142857 0.58571429 0.6 0.61428571 0.62857143 0.64285714 0.65714286 0.67142857 0.68571429 0.7 0.71428571 0.72857143 0.74285714 0.75714286 0.77142857 0.78571429 0.8 0.81428571 0.82857143 0.84285714 0.85714286 0.87142857 0.88571429 0.9 0.91428571 0.92857143 0.94285714 0.95714286 0.97142857 0.98571429 1 1 1 1 1 1
  arc A30 (8.436577, 3.134352) -> (8.181883, 3.749239) centre (0, 0) ccw
  spline S15 degree 5 poles (6.576327, 3.642161) (6.580125, 3.644257) (6.587773, 3.64834) (6.599403, 3.654137) (6.615212, 3.661242) (6.635392, 3.669269) (6.655881, 3.676674) (6.676569, 3.683691) (6.697374, 3.690493) (6.718261, 3.697149) (6.739229, 3.703656) (6.760296, 3.709965) (6.781487, 3.716015) (6.802821, 3.721762) (6.824297, 3.727201) (6.845905, 3.732353) (6.867628, 3.737253) (6.889448, 3.741942) (6.91135, 3.746447) (6.933329, 3.750779) (6.955385, 3.754937) (6.977519, 3.758912) (6.999737, 3.762695) (7.022039, 3.766279) (7.044424, 3.769666) (7.066888, 3.772862) (7.089427, 3.775875) (7.112037, 3.778713) (7.134714, 3.781383) (7.157456, 3.783889) (7.180261, 3.78623) (7.20313, 3.788407) (7.226061, 3.790419) (7.249054, 3.792266) (7.272109, 3.79395) (7.295222, 3.795472) (7.318393, 3.796835) (7.341619, 3.798041) (7.3649, 3.799094) (7.388233, 3.799994) (7.411618, 3.800741) (7.435054, 3.801338) (7.458541, 3.801784) (7.482076, 3.80208) (7.505659, 3.802228) (7.52929, 3.802228) (7.552966, 3.802081) (7.576688, 3.801789) (7.600453, 3.801352) (7.624262, 3.800772) (7.648112, 3.800049) (7.672004, 3.799184) (7.695937, 3.798177) (7.719909, 3.79703) (7.74392, 3.795742) (7.767969, 3.794315) (7.792055, 3.792749) (7.816177, 3.791045) (7.840335, 3.789203) (7.864528, 3.787225) (7.888755, 3.78511) (7.913015, 3.782859) (7.937309, 3.780473) (7.961634, 3.777952) (7.98599, 3.775296) (8.010377, 3.772507) (8.034793, 3.769584) (8.059237, 3.766529) (8.08371, 3.763341) (8.108211, 3.760021) (8.132739, 3.756569) (8.152383, 3.753703) (8.167128, 3.751494) (8.176964, 3.749995) (8.181883, 3.749239) knots 0 0 0 0 0 0 0.01428571 0.02857143 0.04285714 0.05714286 0.07142857 0.08571429 0.1 0.11428571 0.12857143 0.14285714 0.15714286 0.17142857 0.18571429 0.2 0.21428571 0.22857143 0.24285714 0.25714286 0.27142857 0.28571429 0.3 0.31428571 0.32857143 0.34285714 0.35714286 0.37142857 0.38571429 0.4 0.41428571 0.42857143 0.44285714 0.45714286 0.47142857 0.48571429 0.5 0.51428571 0.52857143 0.54285714 0.55714286 0.57142857 0.58571429 0.6 0.61428571 0.62857143 0.64285714 0.65714286 0.67142857 0.68571429 0.7 0.71428571 0.72857143 0.74285714 0.75714286 0.77142857 0.78571429 0.8 0.81428571 0.82857143 0.84285714 0.85714286 0.87142857 0.88571429 0.9 0.91428571 0.92857143 0.94285714 0.95714286 0.97142857 0.98571429 1 1 1 1 1 1
  line L15 (6.576327, 3.642161) -> (6.075954, 3.365981)
  arc A31 (5.807222, 3.439167) -> (6.075954, 3.365981) centre (5.979309, 3.54108) ccw
  arc A32 (5.807222, 3.439167) -> (5.399704, 4.049062) centre (0, 0) ccw
  arc A33 (5.434928, 4.325344) -> (5.399704, 4.049062) centre (5.559714, 4.169048) ccw
  line L16 (5.434928, 4.325344) -> (5.88157, 4.68194)
  spline S16 degree 5 poles (5.88157, 4.68194) (5.88496, 4.684646) (5.891658, 4.690149) (5.901465, 4.698676) (5.914079, 4.710563) (5.929217, 4.726135) (5.943899, 4.742229) (5.958299, 4.758658) (5.972545, 4.775276) (5.986688, 4.792027) (6.000723, 4.808908) (6.014614, 4.825957) (6.028313, 4.84322) (6.041787, 4.86073) (6.05503, 4.87849) (6.068059, 4.896482) (6.080899, 4.914676) (6.093581, 4.93304) (6.106125, 4.951551) (6.118538, 4.970199) (6.13082, 4.988985) (6.142963, 5.007914) (6.15496, 5.026993) (6.166806, 5.046226) (6.178501, 5.06561) (6.190051, 5.085142) (6.20146, 5.104812) (6.212734, 5.124615) (6.22388, 5.144544) (6.234897, 5.164595) (6.245788, 5.184769) (6.25655, 5.205064) (6.267184, 5.225479) (6.27769, 5.246016) (6.288068, 5.266671) (6.298319, 5.287442) (6.308445, 5.308327) (6.318449, 5.329324) (6.32833, 5.35043) (6.338091, 5.371643) (6.347731, 5.392962) (6.35725, 5.414386) (6.36665, 5.435913) (6.375931, 5.457544) (6.385092, 5.479276) (6.394135, 5.501107) (6.40306, 5.523038) (6.411868, 5.545065) (6.420559, 5.567189) (6.429134, 5.589407) (6.437594, 5.611719) (6.445937, 5.634123) (6.454166, 5.656619) (6.462279, 5.679205) (6.470278, 5.701881) (6.478163, 5.724646) (6.485934, 5.747498) (6.49359, 5.770436) (6.501134, 5.79346) (6.508564, 5.816568) (6.515881, 5.839761) (6.523086, 5.863036) (6.530178, 5.886393) (6.537157, 5.909831) (6.544025, 5.93335) (6.55078, 5.956947) (6.557424, 5.980623) (6.563955, 6.004376) (6.570375, 6.028206) (6.576684, 6.052112) (6.582882, 6.076094) (6.587751, 6.09534) (6.591353, 6.109808) (6.593732, 6.119468) (6.594916, 6.124302) knots 0 0 0 0 0 0 0.01428571 0.02857143 0.04285714 0.05714286 0.07142857 0.08571429 0.1 0.11428571 0.12857143 0.14285714 0.15714286 0.17142857 0.18571429 0.2 0.21428571 0.22857143 0.24285714 0.25714286 0.27142857 0.28571429 0.3 0.31428571 0.32857143 0.34285714 0.35714286 0.37142857 0.38571429 0.4 0.41428571 0.42857143 0.44285714 0.45714286 0.47142857 0.48571429 0.5 0.51428571 0.52857143 0.54285714 0.55714286 0.57142857 0.58571429 0.6 0.61428571 0.62857143 0.64285714 0.65714286 0.67142857 0.68571429 0.7 0.71428571 0.72857143 0.74285714 0.75714286 0.77142857 0.78571429 0.8 0.81428571 0.82857143 0.84285714 0.85714286 0.87142857 0.88571429 0.9 0.91428571 0.92857143 0.94285714 0.95714286 0.97142857 0.98571429 1 1 1 1 1 1
  arc A34 (6.594916, 6.124302) -> (6.124302, 6.594916) centre (0, 0) ccw
  spline S17 degree 5 poles (4.68194, 5.88157) (4.684646, 5.88496) (4.690149, 5.891658) (4.698676, 5.901465) (4.710563, 5.914079) (4.726135, 5.929217) (4.742229, 5.943899) (4.758658, 5.958299) (4.775276, 5.972545) (4.792027, 5.986688) (4.808908, 6.000723) (4.825957, 6.014614) (4.84322, 6.028313) (4.86073, 6.041787) (4.87849, 6.05503) (4.896482, 6.068059) (4.914676, 6.080899) (4.93304, 6.093581) (4.951551, 6.106125) (4.970199, 6.118538) (4.988985, 6.13082) (5.007914, 6.142963) (5.026993, 6.15496) (5.046226, 6.166806) (5.06561, 6.178501) (5.085142, 6.190051) (5.104812, 6.20146) (5.124615, 6.212734) (5.144544, 6.22388) (5.164595, 6.234897) (5.184769, 6.245788) (5.205064, 6.25655) (5.225479, 6.267184) (5.246016, 6.27769) (5.266671, 6.288068) (5.287442, 6.298319) (5.308327, 6.308445) (5.329324, 6.318449) (5.35043, 6.32833) (5.371643, 6.338091) (5.392962, 6.347731) (5.414386, 6.35725) (5.435913, 6.36665) (5.457544, 6.375931) (5.479276, 6.385092) (5.501107, 6.394135) (5.523038, 6.40306) (5.545065, 6.411868) (5.567189, 6.420559) (5.589407, 6.429134) (5.611719, 6.437594) (5.634123, 6.445937) (5.656619, 6.454166) (5.679205, 6.462279) (5.701881, 6.470278) (5.724646, 6.478163) (5.747498, 6.485934) (5.770436, 6.49359) (5.79346, 6.501134) (5.816568, 6.508564) (5.839761, 6.515881) (5.863036, 6.523086) (5.886393, 6.530178) (5.909831, 6.537157) (5.93335, 6.544025) (5.956947, 6.55078) (5.980623, 6.557424) (6.004376, 6.563955) (6.028206, 6.570375) (6.052112, 6.576684) (6.076094, 6.582882) (6.09534, 6.587751) (6.109808, 6.591353) (6.119468, 6.593732) (6.124302, 6.594916) knots 0 0 0 0 0 0 0.01428571 0.02857143 0.04285714 0.05714286 0.07142857 0.08571429 0.1 0.11428571 0.12857143 0.14285714 0.15714286 0.17142857 0.18571429 0.2 0.21428571 0.22857143 0.24285714 0.25714286 0.27142857 0.28571429 0.3 0.31428571 0.32857143 0.34285714 0.35714286 0.37142857 0.38571429 0.4 0.41428571 0.42857143 0.44285714 0.45714286 0.47142857 0.48571429 0.5 0.51428571 0.52857143 0.54285714 0.55714286 0.57142857 0.58571429 0.6 0.61428571 0.62857143 0.64285714 0.65714286 0.67142857 0.68571429 0.7 0.71428571 0.72857143 0.74285714 0.75714286 0.77142857 0.78571429 0.8 0.81428571 0.82857143 0.84285714 0.85714286 0.87142857 0.88571429 0.9 0.91428571 0.92857143 0.94285714 0.95714286 0.97142857 0.98571429 1 1 1 1 1 1
  line L17 (4.68194, 5.88157) -> (4.325344, 5.434928)
  arc A35 (4.049062, 5.399704) -> (4.325344, 5.434928) centre (4.169048, 5.559714) ccw
  arc A36 (4.049062, 5.399704) -> (3.439167, 5.807222) centre (0, 0) ccw
  arc A37 (3.365981, 6.075954) -> (3.439167, 5.807222) centre (3.54108, 5.979309) ccw
  line L18 (3.365981, 6.075954) -> (3.642161, 6.576327)
  spline S18 degree 5 poles (3.642161, 6.576327) (3.644257, 6.580125) (3.64834, 6.587773) (3.654137, 6.599403) (3.661242, 6.615212) (3.669269, 6.635392) (3.676674, 6.655881) (3.683691, 6.676569) (3.690493, 6.697374) (3.697149, 6.718261) (3.703656, 6.739229) (3.709965, 6.760296) (3.716015, 6.781487) (3.721762, 6.802821) (3.727201, 6.824297) (3.732353, 6.845905) (3.737253, 6.867628) (3.741942, 6.889448) (3.746447, 6.91135) (3.750779, 6.933329) (3.754937, 6.955385) (3.758912, 6.977519) (3.762695, 6.999737) (3.766279, 7.022039) (3.769666, 7.044424) (3.772862, 7.066888) (3.775875, 7.089427) (3.778713, 7.112037) (3.781383, 7.134714) (3.783889, 7.157456) (3.78623, 7.180261) (3.788407, 7.20313) (3.790419, 7.226061) (3.792266, 7.249054) (3.79395, 7.272109) (3.795472, 7.295222) (3.796835, 7.318393) (3.798041, 7.341619) (3.799094, 7.3649) (3.799994, 7.388233) (3.800741, 7.411618) (3.801338, 7.435054) (3.801784, 7.458541) (3.80208, 7.482076) (3.802228, 7.505659) (3.802228, 7.52929) (3.802081, 7.552966) (3.801789, 7.576688) (3.801352, 7.600453) (3.800772, 7.624262) (3.800049, 7.648112) (3.799184, 7.672004) (3.798177, 7.695937) (3.79703, 7.719909) (3.795742, 7.74392) (3.794315, 7.767969) (3.792749, 7.792055) (3.791045, 7.816177) (3.789203, 7.840335) (3.787225, 7.864528) (3.78511, 7.888755) (3.782859, 7.913015) (3.780473, 7.937309) (3.777952, 7.961634) (3.775296, 7.98599) (3.772507, 8.010377) (3.769584, 8.034793) (3.766529, 8.059237) (3.763341, 8.08371) (3.760021, 8.108211) (3.756569, 8.132739) (3.753703, 8.152383) (3.751494, 8.167128) (3.749995, 8.176964) (3.749239, 8.181883) knots 0 0 0 0 0 0 0.01428571 0.02857143 0.04285714 0.05714286 0.07142857 0.08571429 0.1 0.11428571 0.12857143 0.14285714 0.15714286 0.17142857 0.18571429 0.2 0.21428571 0.22857143 0.24285714 0.25714286 0.27142857 0.28571429 0.3 0.31428571 0.32857143 0.34285714 0.35714286 0.37142857 0.38571429 0.4 0.41428571 0.42857143 0.44285714 0.45714286 0.47142857 0.48571429 0.5 0.51428571 0.52857143 0.54285714 0.55714286 0.57142857 0.58571429 0.6 0.61428571 0.62857143 0.64285714 0.65714286 0.67142857 0.68571429 0.7 0.71428571 0.72857143 0.74285714 0.75714286 0.77142857 0.78571429 0.8 0.81428571 0.82857143 0.84285714 0.85714286 0.87142857 0.88571429 0.9 0.91428571 0.92857143 0.94285714 0.95714286 0.97142857 0.98571429 1 1 1 1 1 1
  arc A38 (3.749239, 8.181883) -> (3.134352, 8.436577) centre (0, 0) ccw